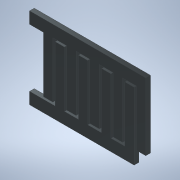
# Autodesk Inventor part: sensor-0001-001
Saved by Autodesk Inventor 2020.1 (Build 241239000, 239)
## iProperties
Created: 2024-03-23
Part Number: sensor-0001-001
Material: Iron, Cast
Document SubType Name: Modeling
Designer: MiguelBarbosa
Density: 7.15 g/cm^3
Appearance: Iron Gray
Author: MiguelBarbosa
Autodesk Inventor part; units mm, degrees
ref_plane "YZ Plane" through (0, 0, 0) normal (1, 0, 0) x (0, 1, 0)
ref_plane "XZ Plane" through (0, 0, 0) normal (0, 1, 0) x (-1, 0, 0)
ref_plane "XY Plane" through (0, 0, 0) normal (0, 0, 1) x (1, 0, 0)
sketch "Sketch2" plane through (0, 0, 0) normal (0, 0, 1) x (1, 0, 0)
  line L0 (-25, -17.5) -> (25, -17.5) construction
  line L1 (25, -17.5) -> (25, 17.5) construction
  line L2 (25, 17.5) -> (-25, 17.5)
  line L3 (-25, 17.5) -> (-25, -17.5) construction
  line L4 (-25, -17.5) -> (25, 17.5) construction
  line L5 (25, -17.5) -> (-25, 17.5) construction
  line L6 (-25, 17.5) -> (-25, 12.5)
  line L7 (25, 17.5) -> (25, -11.5)
  line L8 (25, -11.5) -> (21, -11.5)
  line L9 (21, -11.5) -> (21, 12.5)
  line L10 (21, 12.5) -> (15, 12.5)
  line L11 (15, 12.5) -> (15, -11.5)
  line L12 (15, -11.5) -> (11, -11.5)
  line L13 (11, -11.5) -> (11, 12.5)
  line L14 (11, 12.5) -> (5, 12.5)
  line L15 (5, 12.5) -> (5, -11.5)
  line L16 (5, -11.5) -> (1, -11.5)
  line L17 (1, -11.5) -> (1, 12.5)
  line L18 (1, 12.5) -> (-5, 12.5)
  line L19 (-5, 12.5) -> (-5, -11.5)
  line L20 (-5, -11.5) -> (-9, -11.5)
  line L21 (-9, -11.5) -> (-9, 12.5)
  line L22 (-9, 12.5) -> (-15, 12.5)
  line L23 (-15, 12.5) -> (-15, -11.5)
  line L24 (-15, -11.5) -> (-19, -11.5)
  line L25 (-19, -11.5) -> (-19, 12.5)
  line L26 (-19, 12.5) -> (-25, 12.5)
  line L27 (-25, -17.5) -> (20, -17.5)
  line L28 (20, 11.5) -> (20, -17.5)
  line L29 (20, 11.5) -> (16, 11.5)
  line L30 (16, 11.5) -> (16, -12.5)
  line L31 (16, -12.5) -> (10, -12.5)
  line L32 (10, -12.5) -> (10, 11.5)
  line L33 (10, 11.5) -> (6, 11.5)
  line L34 (6, 11.5) -> (6, -12.5)
  line L35 (6, -12.5) -> (0, -12.5)
  line L36 (0, -12.5) -> (0, 11.5)
  line L37 (0, 11.5) -> (-4, 11.5)
  line L38 (-4, 11.5) -> (-4, -12.5)
  line L39 (-4, -12.5) -> (-10, -12.5)
  line L40 (-10, -12.5) -> (-10, 11.5)
  line L41 (-10, 11.5) -> (-14, 11.5)
  line L42 (-14, 11.5) -> (-14, -12.5)
  line L43 (-14, -12.5) -> (-25, -12.5)
  line L44 (-25, -12.5) -> (-25, -17.5)
  point P0 (0, 0)
  dimension "d17" = 50
  dimension "d18" = 35
  dimension "d19" = 5
  dimension "d21" = 4
  dimension "d22" = 6
  dimension "d23" = 1
  dimension "d24" = 1
  dimension "d25" = 1
  dimension "d26" = 1
  dimension "d27" = 5
  constraints: 90 end point, 23 equal length, 20 perpendicular, 10 point on line, 8 horizontal, 7 vertical, 2 midpoint, 2 parallel, 1 collinear, 1 horizontal alignment
  measures "d17" distance of L1.end L2.end
  measures "d18" distance of L2.end L0.start
  measures "d19" distance of L2.end L6.end
  measures "d21" distance of L7.end L8.end
  measures "d22" distance of L9.end L10.end
  measures "d23" distance between parallel lines of L9 L28
  measures "d24" distance between parallel lines of L10 L29
  measures "d25" distance between parallel lines of L11 L30
  measures "d26" distance between parallel lines of L31 L12
  measures "d27" distance of L43.end L0.start
extrude "Extrusion2" add sketch "Sketch2" along normal mid plane 2
sketch "Sketch1" plane through (0, 0, 0) normal (0, 0, 1) x (1, 0, 0)
  line L0 (-60, 75) -> (60, 75)
  line L1 (60, 75) -> (60, -75) construction
  line L2 (60, -75) -> (-60, -75) construction
  line L3 (-60, -75) -> (-60, 75) construction
  line L4 (-60, 75) -> (-60, 65)
  line L5 (-60, 65) -> (-30, 65)
  line L6 (-30, 65) -> (-30, -55)
  line L7 (-30, -55) -> (-21.7778, -55)
  line L8 (-21.7778, -55) -> (-21.7778, 65)
  line L9 (-21.7778, 65) -> (-9.5556, 65)
  line L10 (-9.5556, 65) -> (-9.5556, -55)
  line L11 (-9.5556, -55) -> (-1.3333, -55)
  line L12 (-1.3333, -55) -> (-1.3333, 65)
  line L13 (-1.3333, 65) -> (10.8889, 65)
  line L14 (10.8889, 65) -> (10.8889, -55)
  line L15 (10.8889, -55) -> (19.1111, -55)
  line L16 (19.1111, -55) -> (19.1111, 65)
  line L17 (19.1111, 65) -> (31.3333, 65)
  line L18 (31.3333, 65) -> (31.3333, -55)
  line L19 (31.3333, -55) -> (39.5556, -55)
  line L20 (39.5556, -55) -> (39.5556, 65)
  line L21 (39.5556, 65) -> (51.7778, 65)
  line L22 (60, 75) -> (60, -55)
  line L23 (51.7778, 65) -> (51.7778, -55)
  line L24 (51.7778, -55) -> (60, -55)
  line L25 (-60, -75) -> (-60, -65)
  line L26 (-60, -65) -> (-19.7778, -65)
  line L27 (-60, -75) -> (49.7778, -75)
  line L28 (-19.7778, -65) -> (-19.7778, 63)
  line L29 (-19.7778, 63) -> (-11.5556, 63)
  line L30 (-11.5556, 63) -> (-11.5556, -65)
  line L31 (-11.5556, -65) -> (0.6667, -65)
  line L32 (0.6667, -65) -> (0.6667, 63)
  line L33 (0.6667, 63) -> (8.8889, 63)
  line L34 (8.8889, 63) -> (8.8889, -65)
  line L35 (8.8889, -65) -> (21.1111, -65)
  line L36 (21.1111, -65) -> (21.1111, 63)
  line L37 (21.1111, 63) -> (29.3333, 63)
  line L38 (29.3333, 63) -> (29.3333, -65)
  line L39 (29.3333, -65) -> (41.5556, -65)
  line L40 (41.5556, -65) -> (41.5556, 63)
  line L41 (41.5556, 63) -> (49.7778, 63)
  line L42 (49.7778, 63) -> (49.7778, -75)
  point P0 (0, 0)
  point P1 (0, 75)
  point P2 (-60, 0)
  point P3 (-15.6667, 63)
  point P4 (-15.6667, 65)
  point P5 (-5.4444, -55)
  point P6 (-5.4444, -65)
  point P7 (45.6667, 63)
  point P8 (45.6667, 65)
  point P9 (4.7778, 63)
  point P10 (4.7778, 65)
  point P11 (25.2222, 63)
  point P12 (25.2222, 65)
  point P13 (15, -55)
  point P14 (15, -65)
  point P15 (35.4444, -55)
  point P16 (35.4444, -65)
  dimension "d5" = 150
  dimension "d7" = 10
  dimension "d9" = 120
  dimension "d11" = 2
  dimension "d12" = 2
  dimension "d13" = 120
  dimension "d14" = 30
  constraints: 86 end point, 22 equal length, 16 midpoint, 15 horizontal, 11 perpendicular, 8 vertical alignment, 7 vertical, 6 parallel, 4 point on line, 2 horizontal alignment
  measures "d5" distance of L2.end L0.start
  measures "d7" distance of L0.start L4.end
  measures "d9" distance of L5.end L6.end
  measures "d11" distance between parallel lines of L8 L28
  measures "d12" distance between parallel lines of L9 L29
  measures "d13" distance of L0.start L0.end
  measures "d14" distance of L4.end L5.end
equation "\"d24\" = d23"
equation "\"d25\" = d23"
equation "\"d26\" = d23"
equation "\"d27\" = d19"
equation "\"d12\" = d11"
body "Solid1"
body "Solid2"
